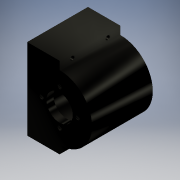
# Autodesk Inventor part: BracketHusillo
Saved by Autodesk Inventor 2018 (Build 220112000, 112)
## iProperties
Created: 2018-01-14
Part Number: BracketHusillo
Material: Genérico
Document SubType Name: Modeling
Designer: Carlos
Density: 1 g/cm^3
Appearance: Gris plomo
Author: Carlos
Autodesk Inventor part; units mm, degrees
ref_plane "YZ Plane" through (0, 0, 0) normal (1, 0, 0) x (0, 1, 0)
ref_plane "XZ Plane" through (0, 0, 0) normal (0, 1, 0) x (-1, 0, 0)
ref_plane "XY Plane" through (0, 0, 0) normal (0, 0, 1) x (1, 0, 0)
sketch "Boceto1" plane through (0, 0, 0) normal (0, 1, 0) x (-1, 0, 0)
  circle A0 centre (0, 0) radius 26
  circle A1 centre (0, 0) radius 32
  line L0 (0, 40) -> (32, 40)
  line L1 (32, 40) -> (32, -40)
  line L2 (32, -40) -> (0, -40)
  line L3 (0, -40) -> (0, 40)
  dimension "d0" = 52
  dimension "d1" = 64
  dimension "d2" = 40
  dimension "d3" = 80
  dimension "d4" = 32
  dimension "d5" = 32
  constraints: 8 end point, 2 centre point, 2 coincident, 2 parallel, 1 horizontal, 1 perpendicular
  measures "d0" diameter of A0
  measures "d1" diameter of A1
  measures "d2" distance from line of L0 point (0, 0)
  measures "d3" distance of L0.end L1.end
  measures "d4" distance of L1.end L2.end
  measures "d5" distance from line of L1 point (0, 0)
extrude "Extrusión1" add sketch "Boceto1" along normal blind 67
sketch "Boceto2" plane through (0, 67, 0) normal (0, 1, 0) x (1, 0, 0)
  circle A0 centre (0, 0) radius 26
  dimension "d8" = 52
  constraints: 1 centre point, 1 coincident
  measures "d8" diameter of A0
hole "Agujero1" at (0, 67, 0) direction (0, -1, 0) diameter 52 depth 60
sketch "Boceto3" plane through (0, 0, 0) normal (0, -1, 0) x (1, 0, 0)
  circle A0 centre (0, 0) radius 13
  dimension "d16" = 26
  constraints: 1 centre point, 1 coincident
  measures "d16" diameter of A0
hole "Agujero2" at (0, 0, 0) direction (0, 1, 0) diameter 26 depth 60
sketch "Boceto4" plane through (0, 0, 0) normal (0, -1, 0) x (1, 0, 0)
  circle A0 centre (0, 0) radius 17.75
  circle A1 centre (17.75, 0) radius 2
  circle A2 centre (0, -17.75) radius 2
  circle A3 centre (-17.75, 0) radius 2
  circle A4 centre (0, 17.75) radius 2
  dimension "d24" = 35.5
  dimension "d25" = 4
  dimension "d26" = 4
  dimension "d27" = 4
  dimension "d28" = 4
  constraints: 5 centre point, 4 point on circle, 1 coincident
  measures "d24" diameter of A0
  measures "d25" diameter of A1
  measures "d26" diameter of A2
  measures "d27" diameter of A4
  measures "d28" diameter of A3
hole "Agujero3" at (17.75, 0, 0) at (0, 0, -17.75) at (-17.75, 0, 0) at (0, 0, 17.75) direction (0, 1, 0) diameter 4 depth 60
sketch "Boceto5" plane through (0, 67, 0) normal (0, 1, 0) x (1, 0, 0)
  point P0 (0, 0)
  point P1 (0, 0)
  constraints: 1 coincident
hole "Agujero4" at (0, 67, 0) direction (0, -1, 0) diameter 200 depth 7
sketch "Boceto6" plane through (-32, 0, -40) normal (-1, 0, 0) x (0, 0, 1)
  line L0 (4, 12.5) -> (76, 12.5)
  line L1 (76, 12.5) -> (76, 47.5)
  line L2 (76, 47.5) -> (4, 47.5)
  line L3 (4, 47.5) -> (4, 12.5)
  line L4 (4, 12.5) -> (76, 47.5) construction
  line L5 (76, 12.5) -> (4, 47.5) construction
  line L6 (80, 0) -> (80, 60) projected
  line L7 (80, 60) -> (0, 60) projected
  circle A0 centre (4, 47.5) radius 2
  circle A1 centre (76, 47.5) radius 2
  circle A2 centre (76, 12.5) radius 2
  circle A3 centre (4, 12.5) radius 2
  point P0 (40, 0)
  point P1 (40, 30)
  dimension "d43" = 35
  dimension "d44" = 40
  dimension "d45" = 30
  dimension "d46" = 72
  dimension "d47" = 4
  dimension "d48" = 4
  dimension "d49" = 4
  dimension "d50" = 4
  constraints: 12 end point, 4 centre point, 4 coincident, 2 midpoint, 2 parallel, 1 horizontal, 1 perpendicular
  measures "d43" distance of L0.end L1.end
  measures "d44" distance from line of L6 point (40, 30)
  measures "d45" distance from line of L7 point (40, 30)
  measures "d46" distance of L0.start L0.end
  measures "d47" diameter of A0
  measures "d48" diameter of A1
  measures "d49" diameter of A2
  measures "d50" diameter of A3
hole "Agujero5" at (-32, 47.5, -36) at (-32, 12.5, -36) at (-32, 12.5, 36) at (-32, 47.5, 36) direction (1, 0, 0) diameter 4 depth 32
